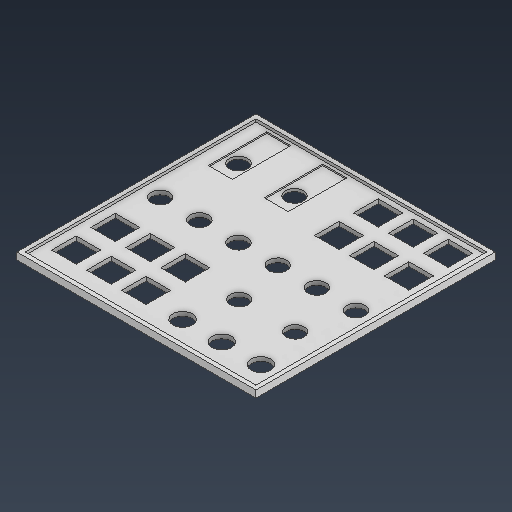
# Autodesk Inventor part: Faceplate
Saved by Autodesk Inventor 2025.3 (Build 293356000, 356)
## iProperties
Created: 2025-09-08
Part Number: Faceplate
Material: Generic
Document SubType Name: Modeling
Designer: tolga
Density: 1 g/cm^3
Appearance: Default
Author: tolga
Autodesk Inventor part; units mm, degrees
ref_plane "YZ Plane" through (0, 0, 0) normal (1, 0, 0) x (0, 1, 0)
ref_plane "XZ Plane" through (0, 0, 0) normal (0, 1, 0) x (-1, 0, 0)
ref_plane "XY Plane" through (0, 0, 0) normal (0, 0, 1) x (1, 0, 0)
sketch "Sketch1" plane through (0, 0, 0) normal (0, 1, 0) x (-1, 0, 0)
  line L0 (0, 0) -> (-171, 0)
  line L1 (-171, 0) -> (-171, -171)
  line L2 (-171, -171) -> (0, -171)
  line L3 (0, -171) -> (0, 0)
  dimension "d0" = 171
  dimension "d1" = 171
  constraints: 8 end point, 2 parallel, 1 horizontal, 1 perpendicular
  measures "d0" distance of L2.end L1.end
  measures "d1" distance of L1.end L0.end
extrude "Extrusion1" add sketch "Sketch1" along normal blind 3
sketch "Sketch2" plane through (0, 3, 0) normal (0, 1, 0) x (1, 0, 0)
  line L0 (171, 0) -> (171, 171) projected
  line L1 (171, 171) -> (0, 171) projected
  line L2 (0, 171) -> (0, 0) projected
  line L3 (0, 0) -> (171, 0) projected
  line L4 (3, 3) -> (3, 168)
  line L5 (3, 168) -> (168, 168)
  line L6 (168, 168) -> (168, 3)
  line L7 (168, 3) -> (3, 3)
  dimension "d98" = 165
  constraints: 8 end point, 3 other
  measures "d98" distance between parallel lines of L6 L4
extrude "Extrusion2" add sketch "Sketch2" along normal blind 2
sketch "Sketch3" plane through (0, 3, 0) normal (0, 1, 0) x (1, 0, 0)
  line L0 (3, 3) -> (168, 3) construction
  line L1 (168, 3) -> (168, 168) construction
  line L2 (168, 168) -> (3, 168) construction
  line L3 (3, 168) -> (3, 3) construction
  line L4 (4, 64) -> (82, 64) construction
  line L5 (82, 64) -> (82, 4) construction
  line L6 (82, 4) -> (4, 4) construction
  line L7 (4, 4) -> (4, 64) construction
  line L8 (89, 107) -> (167, 107) construction
  line L9 (167, 107) -> (167, 167) construction
  line L10 (167, 167) -> (89, 167) construction
  line L11 (89, 167) -> (89, 107) construction
  line L12 (4, 167) -> (79, 167) construction
  line L13 (79, 167) -> (79, 102) construction
  line L14 (4, 72) -> (4, 167) construction
  line L15 (4, 72) -> (167, 72) construction
  line L16 (167, 72) -> (167, 102) construction
  line L17 (167, 102) -> (79, 102) construction
  line L18 (87, 67) -> (167, 67) construction
  line L19 (167, 67) -> (167, 37) construction
  line L20 (167, 37) -> (87, 37) construction
  line L21 (87, 37) -> (87, 67) construction
  line L22 (87, 32) -> (167, 32) construction
  line L23 (167, 32) -> (167, 7) construction
  line L24 (167, 7) -> (87, 7) construction
  line L25 (87, 7) -> (87, 32) construction
  line L26 (9.25, 33.15) -> (26.75, 33.15)
  line L27 (26.75, 33.15) -> (26.75, 15.65)
  line L28 (26.75, 15.65) -> (9.25, 15.65)
  line L29 (9.25, 15.65) -> (9.25, 33.15)
  line L30 (9.25, 61.15) -> (26.75, 61.15)
  line L31 (9.25, 43.65) -> (9.25, 61.15)
  line L32 (26.75, 43.65) -> (9.25, 43.65)
  line L33 (26.75, 61.15) -> (26.75, 43.65)
  line L34 (34.25, 33.15) -> (51.75, 33.15)
  line L35 (34.25, 15.65) -> (34.25, 33.15)
  line L36 (51.75, 15.65) -> (34.25, 15.65)
  line L37 (51.75, 33.15) -> (51.75, 15.65)
  line L38 (34.25, 61.15) -> (51.75, 61.15)
  line L39 (34.25, 43.65) -> (34.25, 61.15)
  line L40 (51.75, 43.65) -> (34.25, 43.65)
  line L41 (51.75, 61.15) -> (51.75, 43.65)
  line L42 (59.25, 33.15) -> (76.75, 33.15)
  line L43 (59.25, 15.65) -> (59.25, 33.15)
  line L44 (76.75, 15.65) -> (59.25, 15.65)
  line L45 (76.75, 33.15) -> (76.75, 15.65)
  line L46 (59.25, 61.15) -> (76.75, 61.15)
  line L47 (59.25, 43.65) -> (59.25, 61.15)
  line L48 (76.75, 43.65) -> (59.25, 43.65)
  line L49 (76.75, 61.15) -> (76.75, 43.65)
  line L50 (9.25, 61.15) -> (9.25, 15.65) construction
  line L51 (9.25, 61.15) -> (76.75, 61.15) construction
  line L52 (94.25, 136.15) -> (111.75, 136.15)
  line L53 (111.75, 136.15) -> (111.75, 118.65)
  line L54 (111.75, 118.65) -> (94.25, 118.65)
  line L55 (94.25, 118.65) -> (94.25, 136.15)
  line L56 (94.25, 164.15) -> (111.75, 164.15)
  line L57 (94.25, 146.65) -> (94.25, 164.15)
  line L58 (111.75, 146.65) -> (94.25, 146.65)
  line L59 (111.75, 164.15) -> (111.75, 146.65)
  line L60 (119.25, 136.15) -> (136.75, 136.15)
  line L61 (119.25, 118.65) -> (119.25, 136.15)
  line L62 (136.75, 118.65) -> (119.25, 118.65)
  line L63 (136.75, 136.15) -> (136.75, 118.65)
  line L64 (119.25, 164.15) -> (136.75, 164.15)
  line L65 (119.25, 146.65) -> (119.25, 164.15)
  line L66 (136.75, 146.65) -> (119.25, 146.65)
  line L67 (136.75, 164.15) -> (136.75, 146.65)
  line L68 (144.25, 136.15) -> (161.75, 136.15)
  line L69 (144.25, 118.65) -> (144.25, 136.15)
  line L70 (161.75, 118.65) -> (144.25, 118.65)
  line L71 (161.75, 136.15) -> (161.75, 118.65)
  line L72 (144.25, 164.15) -> (161.75, 164.15)
  line L73 (144.25, 146.65) -> (144.25, 164.15)
  line L74 (161.75, 146.65) -> (144.25, 146.65)
  line L75 (161.75, 164.15) -> (161.75, 146.65)
  line L76 (94.25, 164.15) -> (94.25, 118.65) construction
  line L77 (94.25, 164.15) -> (161.75, 164.15) construction
  circle A0 centre (107, 52) radius 12.5 construction
  circle A1 centre (147, 52) radius 12.5 construction
  circle A2 centre (107, 52) radius 6.4
  circle A3 centre (147, 52) radius 6.4
  circle A4 centre (99, 19.5) radius 8.1 construction
  circle A5 centre (127, 19.5) radius 8.1 construction
  circle A6 centre (155, 19.5) radius 8.1 construction
  circle A7 centre (99, 19.5) radius 7
  circle A8 centre (127, 19.5) radius 7
  circle A9 centre (155, 19.5) radius 7
  circle A10 centre (155.5, 87) radius 6.5
  circle A11 centre (127.5, 87) radius 6.5
  circle A12 centre (99.5, 87) radius 6.5
  circle A13 centre (71.5, 87) radius 6.5
  circle A14 centre (43.5, 87) radius 6.5
  circle A15 centre (15.5, 87) radius 6.5
  circle A16 centre (61.5, 137) radius 6.5
  circle A17 centre (21.5, 137) radius 6.5
  point P0 (0, 0)
  point P1 (4, 34)
  point P2 (43, 61.15)
  point P3 (43, 64)
  point P4 (18, 43.65)
  point P5 (26.75, 52.4)
  point P6 (128, 164.15)
  point P7 (103, 146.65)
  point P8 (111.75, 155.4)
  point P9 (128, 164.15)
  point P10 (128, 107)
  point P11 (87, 52)
  point P12 (167, 19.5)
  point P13 (167, 87)
  point P14 (79, 134.5)
  point P15 (9.25, 24.4)
  point P16 (94.25, 127.4)
  dimension "d7" = 1
  dimension "d8" = 1
  dimension "d9" = 60
  dimension "d10" = 78
  dimension "d11" = 78
  dimension "d12" = 60
  dimension "d13" = 1
  dimension "d14" = 1
  dimension "d15" = 1
  dimension "d16" = 1
  dimension "d17" = 75
  dimension "d19" = 1
  dimension "d20" = 5
  dimension "d21" = 30
  dimension "d22" = 5
  dimension "d23" = 5
  dimension "d24" = 1
  dimension "d27" = 5
  dimension "d28" = 5
  dimension "d29" = 1
  dimension "d30" = 4
  dimension "d31" = 25
  dimension "d32" = 17.5
  dimension "d33" = 17.5
  dimension "d37" = 28
  dimension "d40" = 25
  dimension "d44" = 5.25
  dimension "d45" = 2.85
  dimension "d46" = 14
  dimension "d47" = 11.6
  dimension "d52" = 17.5
  dimension "d53" = 17.5
  dimension "d54" = 28
  dimension "d55" = 25
  dimension "d57" = 30
  dimension "d58" = 80
  dimension "d59" = 25
  dimension "d60" = 25
  dimension "d61" = 20
  dimension "d62" = 40
  dimension "d63" = 12.8
  dimension "d64" = 12.8
  dimension "d67" = 80
  dimension "d68" = 16.2
  dimension "d69" = 16.2
  dimension "d70" = 16.2
  dimension "d71" = 28
  dimension "d72" = 28
  dimension "d73" = 12
  dimension "d74" = 14
  dimension "d75" = 14
  dimension "d76" = 14
  dimension "d77" = 13
  dimension "d80" = 28
  dimension "d85" = 11.5
  dimension "d86" = 163
  dimension "d87" = 65
  dimension "d88" = 95
  dimension "d89" = 88
  dimension "d90" = 13
  dimension "d91" = 13
  dimension "d92" = 30
  dimension "d93" = 40
  dimension "d94" = 17.5
  constraints: 148 end point, 18 centre point, 16 midpoint, 13 parallel, 11 horizontal, 11 perpendicular, 7 horizontal alignment, 6 collinear, 5 coincident, 2 vertical, 2 vertical alignment, 86 other
  measures "d7" distance between parallel lines of L7 L3
  measures "d8" distance between parallel lines of L0 L6
  measures "d9" distance between parallel lines of L6 L4
  measures "d10" distance between parallel lines of L7 L5
  measures "d11" distance of L10.end L9.end
  measures "d12" distance of L9.end L8.end
  measures "d13" distance between parallel lines of L2 L10
  measures "d14" distance between parallel lines of L1 L9
  measures "d15" distance between parallel lines of L2 L12
  measures "d16" distance between parallel lines of L3 L14
  measures "d17" distance between parallel lines of L14 L13
  measures "d19" distance between parallel lines of L1 L16
  measures "d20" distance between parallel lines of L8 L17
  measures "d21" distance between parallel lines of L17 L15
  measures "d22" distance between parallel lines of L15 L18
  measures "d23" distance between parallel lines of L5 L21
  measures "d24" distance between parallel lines of L1 L19
  measures "d27" distance between parallel lines of L5 L25
  measures "d28" distance between parallel lines of L20 L22
  measures "d29" distance between parallel lines of L1 L23
  measures "d30" distance between parallel lines of L0 L24
  measures "d31" distance between parallel lines of L24 L22
  measures "d32" distance of L27.end L28.end
  measures "d33" distance of L26.end L27.end
  measures "d37" distance of L27.end L32.start
  measures "d40" distance of L27.end L36.start
  measures "d44" distance between parallel lines of L7 L31
  measures "d45" distance between parallel lines of L4 L51
  measures "d46" distance from line of L7 point (18, 43.65)
  measures "d47" distance from line of L4 point (26.75, 52.4)
  measures "d52" distance of L53.end L76.end
  measures "d53" distance of L53.start L53.end
  measures "d54" distance of L53.end L58.start
  measures "d55" distance of L53.end L62.start
  measures "d57" distance between parallel lines of L18 L20
  measures "d58" distance between parallel lines of L19 L21
  measures "d59" diameter of A0
  measures "d60" diameter of A1
  measures "d61" distance from line of L21 A0.centre
  measures "d62" distance of A0.centre A1.centre
  measures "d63" diameter of A2
  measures "d64" diameter of A3
  measures "d67" distance between parallel lines of L23 L25
  measures "d68" diameter of A4
  measures "d69" diameter of A5
  measures "d70" diameter of A6
  measures "d71" distance of A5.centre A4.centre
  measures "d72" distance of A6.centre A5.centre
  measures "d73" distance from line of L25 A4.centre
  measures "d74" diameter of A7
  measures "d75" diameter of A8
  measures "d76" diameter of A9
  measures "d77" diameter of A10
  measures "d80" distance of A10.centre A11.centre
  measures "d85" distance from line of L16 A10.centre
  measures "d86" distance of L14.start L15.end
  measures "d87" distance of L12.end L13.end
  measures "d88" distance of L14.start L12.start
  measures "d89" distance of L16.end L13.end
  measures "d90" diameter of A16
  measures "d91" diameter of A17
  measures "d92" distance from line of L12 A17.centre
  measures "d93" distance of A17.centre A16.centre
  measures "d94" horizontal distance of point (79, 134.5) A16.centre
extrude "Extrusion3" cut sketch "Sketch3" against normal up to surface (3 mm away)
sketch "Sketch5" plane through (0, 3, 0) normal (0, 1, 0) x (1, 0, 0)
  circle A0 centre (21.5, 137) radius 6.5 construction
  circle A1 centre (61.5, 137) radius 6.5 construction
  line L0 (12.9, 165.8) -> (30.1, 165.8)
  line L1 (30.1, 165.8) -> (30.1, 124)
  line L2 (30.1, 124) -> (12.9, 124)
  line L3 (12.9, 124) -> (12.9, 165.8)
  line L4 (70.1, 124) -> (52.9, 124)
  line L5 (52.9, 124) -> (52.9, 165.8)
  line L6 (52.9, 165.8) -> (70.1, 165.8)
  line L7 (70.1, 165.8) -> (70.1, 124)
  point P0 (0, 0)
  point P1 (21.5, 165.8)
  point P2 (61.5, 165.8)
  point P3 (61.5, 124)
  point P4 (21.5, 124)
  dimension "d99" = 13
  dimension "d100" = 28.8
  dimension "d101" = 17.2
  dimension "d102" = 17.2
  constraints: 16 end point, 4 midpoint, 4 parallel, 2 horizontal, 2 horizontal alignment, 2 perpendicular, 2 vertical alignment
  measures "d99" distance from line of L2 A0.centre
  measures "d100" distance of point (21.5, 165.8) A0.centre
  measures "d101" distance between parallel lines of L1 L3
  measures "d102" distance between parallel lines of L7 L5
extrude "Extrusion5" cut sketch "Sketch5" against normal blind 1
equation "\"d8\" = d7"
equation "\"d11\" = d10"
equation "\"d12\" = d9"
equation "\"d13\" = d7"
equation "\"d14\" = d7"
equation "\"d15\" = d7"
equation "\"d16\" = d7"
equation "\"d19\" = d7"
equation "\"d24\" = d7"
equation "\"d29\" = d7"
equation "\"d60\" = d59"
equation "\"d61\" = -0.5 * d62 + 0.5 * d58"
equation "\"d64\" = d63"
equation "\"d69\" = d68"
equation "\"d70\" = d68"
equation "\"d72\" = d71"
equation "\"d73\" = -d71 + 0.5 * d67"
equation "\"d75\" = d74"
equation "\"d76\" = d74"
body "Solid1"
